2080_Simple_v4 (Autodesk Fusion 360 design; units mm, degrees)
Autodesk Fusion 360 part; units mm, degrees
(part 1 of 2)
sketch "Sketch1" plane through (0, 0, 0) normal (0, 0, 1) x (1, 0, 0)
  line L0 (33.9, 0.2048) -> (33.9, 2.8393) construction
  line L1 (25.5058, -9.8977) -> (25.5381, -9.8746) construction
  arc A0 (33.1214, 8.5414) -> (33.2628, 8.2) centre (33.2628, 8.4) ccw construction
  line L2 (39.9538, 4.5991) -> (39.9678, 4.6363) construction
  line L3 (39.5, 10) -> (38.5, 10) construction
  line L4 (34.9, 10) -> (34.7917, 9.9987) construction
  line L5 (34.4312, 9.8494) -> (34.4022, 9.8222) construction
  line L6 (25.5381, -9.8746) -> (25.5688, -9.8494) construction
  line L7 (25.5978, -9.8222) -> (26.8786, -8.5414) construction
  line L8 (26.7372, -8.2) -> (24.5, -8.2) construction
  line L9 (-38.2, -5.5) -> (-38.2, -3.2628) construction
  line L10 (25.4721, -9.9187) -> (25.5058, -9.8977) construction
  line L11 (38.2, 5.5) -> (38.2, 3.2628) construction
  line L12 (34.5991, 9.9538) -> (34.563, 9.9374) construction
  line L13 (25.5688, -9.8494) -> (25.5978, -9.8222) construction
  line L14 (39.9987, 4.7917) -> (40, 4.8314) construction
  arc A1 (38.2, 3.2628) -> (38.5414, 3.1214) centre (38.4, 3.2628) ccw construction
  arc A2 (-33.1214, -8.5414) -> (-33.2628, -8.2) centre (-33.2628, -8.4) ccw construction
  line L15 (39.9948, 4.7522) -> (39.9987, 4.7917) construction
  arc A3 (26.8786, -8.5414) -> (26.7372, -8.2) centre (26.7372, -8.4) ccw construction
  line L16 (33.6952, 0) -> (33.9, 0.2048) construction
  line L17 (-34.5279, -9.9187) -> (-34.4942, -9.8977) construction
  line L18 (33.9, -0.207) -> (33.6952, 0) construction
  line L19 (-34.563, -9.9374) -> (-34.5279, -9.9187) construction
  line L20 (39.8977, 4.4942) -> (39.9187, 4.5279) construction
  line L21 (32.8393, -3.9) -> (35.5, -6.5607) construction
  line L22 (39.9187, 4.5279) -> (39.9374, 4.563) construction
  line L23 (39.9793, 4.6743) -> (39.9883, 4.713) construction
  line L24 (39.9374, 4.563) -> (39.9538, 4.5991) construction
  line L25 (39.8222, 4.4022) -> (39.8494, 4.4312) construction
  line L26 (33.6952, 0) -> (33.9, 0.2048) construction
  line L27 (39.8494, 4.4312) -> (39.8746, 4.4619) construction
  line L28 (39.9883, 4.713) -> (39.9948, 4.7522) construction
  line L29 (33.9, 2.8393) -> (36.5607, 5.5) construction
  line L30 (38.5414, 3.1214) -> (39.8222, 4.4022) construction
  line L31 (39.8746, 4.4619) -> (39.8977, 4.4942) construction
  line L32 (39.9678, 4.6363) -> (39.9793, 4.6743) construction
  line L33 (-34.4022, -9.8222) -> (-33.1214, -8.5414) construction
  line L34 (36.5607, 5.5) -> (38.2, 5.5) construction
  line L35 (-34.4312, -9.8494) -> (-34.4022, -9.8222) construction
  line L36 (-34.4619, -9.8746) -> (-34.4312, -9.8494) construction
  line L37 (-39.9883, -4.713) -> (-39.9948, -4.7522) construction
  line L38 (-25.4721, -9.9187) -> (-25.437, -9.9374) construction
  line L39 (-39.9538, -4.5991) -> (-39.9678, -4.6363) construction
  line L40 (-39.9678, -4.6363) -> (-39.9793, -4.6743) construction
  line L41 (25.1, -10) -> (25.2083, -9.9987) construction
  line L42 (25.437, 9.9374) -> (25.4009, 9.9538) construction
  line L43 (26.1, -0.207) -> (26.1, -2.8393) construction
  line L44 (25.4009, 9.9538) -> (25.3637, 9.9678) construction
  circle A4 centre (30, 0) radius 2.1 construction
  line L45 (-39.9948, -4.7522) -> (-39.9987, -4.7917) construction
  line L46 (-25.3637, -9.9678) -> (-25.3257, -9.9793) construction
  line L47 (-39.9793, -4.6743) -> (-39.9883, -4.713) construction
  line L48 (26.1, 0.207) -> (26.307, 0) construction
  line L49 (26.1, -2.8393) -> (22.7, -6.2393) construction
  line L50 (30.1999, 3.9) -> (30, 3.7001) construction
  line L51 (26.8786, 8.5414) -> (25.5978, 9.8222) construction
  arc A5 (26.7372, 8.2) -> (26.8786, 8.5414) centre (26.7372, 8.4) ccw construction
  line L52 (-25.437, -9.9374) -> (-25.4009, -9.9538) construction
  line L53 (22.7, 8.2) -> (22.7, 6.2393) construction
  line L54 (-25.5058, -9.8977) -> (-25.4721, -9.9187) construction
  line L55 (25.3637, 9.9678) -> (25.3257, 9.9793) construction
  line L56 (27.1607, 3.9) -> (24.5, 6.5607) construction
  arc A6 (-38.2, -3.2628) -> (-38.5414, -3.1214) centre (-38.4, -3.2628) ccw construction
  line L57 (22.7, -6.2393) -> (22.7, -8.2) construction
  line L58 (24.5, 8.2) -> (26.7372, 8.2) construction
  line L59 (-25.3257, -9.9793) -> (-25.287, -9.9883) construction
  line L60 (-39.9987, -4.7917) -> (-40, -4.8314) construction
  line L61 (-25.287, -9.9883) -> (-25.2478, -9.9948) construction
  line L62 (-25.2478, -9.9948) -> (-25.2083, -9.9987) construction
  line L63 (-25.4009, -9.9538) -> (-25.3637, -9.9678) construction
  line L64 (34.4942, 9.8977) -> (34.4619, 9.8746) construction
  arc A7 (40, 9.5) -> (39.5, 10) centre (39.5, 9.5) ccw construction
  line L65 (40, 8.5) -> (40, 9.5) construction
  line L66 (34.6363, 9.9678) -> (34.5991, 9.9538) construction
  line L67 (-25.2083, -9.9987) -> (-25.1, -10) construction
  line L68 (-39.9374, -4.563) -> (-39.9538, -4.5991) construction
  line L69 (25.2083, -9.9987) -> (25.2478, -9.9948) construction
  line L70 (-39.9187, -4.5279) -> (-39.9374, -4.563) construction
  line L71 (35.5, 8.2) -> (35.5, 6.5607) construction
  line L72 (25.3257, -9.9793) -> (25.3637, -9.9678) construction
  line L73 (33.2628, 8.2) -> (35.5, 8.2) construction
  line L74 (-39.8222, -4.4022) -> (-39.8494, -4.4312) construction
  line L75 (34.4619, 9.8746) -> (34.4312, 9.8494) construction
  line L76 (34.7522, 9.9948) -> (34.713, 9.9883) construction
  line L77 (-39.8494, -4.4312) -> (-39.8746, -4.4619) construction
  line L78 (34.4022, 9.8222) -> (33.1214, 8.5414) construction
  line L79 (34.563, 9.9374) -> (34.5279, 9.9187) construction
  line L80 (34.6743, 9.9793) -> (34.6363, 9.9678) construction
  line L81 (25.287, -9.9883) -> (25.3257, -9.9793) construction
  line L82 (-40, -4.8314) -> (-40, -8.5) construction
  line L83 (34.713, 9.9883) -> (34.6743, 9.9793) construction
  line L84 (-39.8746, -4.4619) -> (-39.8977, -4.4942) construction
  line L85 (25.3637, -9.9678) -> (25.4009, -9.9538) construction
  line L86 (-38.5414, -3.1214) -> (-39.8222, -4.4022) construction
  line L87 (25.4009, -9.9538) -> (25.437, -9.9374) construction
  arc A8 (-26.7372, -8.2) -> (-26.8786, -8.5414) centre (-26.7372, -8.4) ccw construction
  line L88 (38.5, 10) -> (34.9, 10) construction
  line L89 (34.5279, 9.9187) -> (34.4942, 9.8977) construction
  line L90 (34.7917, 9.9987) -> (34.7522, 9.9948) construction
  line L91 (25.437, -9.9374) -> (25.4721, -9.9187) construction
  line L92 (25.2478, -9.9948) -> (25.287, -9.9883) construction
  line L93 (-39.8977, -4.4942) -> (-39.9187, -4.5279) construction
  line L94 (39.9374, -4.563) -> (39.9187, -4.5279) construction
  line L95 (-40, -8.5) -> (-40, -9.5) construction
  line L96 (30, -3.7001) -> (30.1999, -3.9) construction
  line L97 (22.7, -6.2393) -> (22.7, -8.2) construction
  line L98 (24.5, -6.5607) -> (27.1607, -3.9) construction
  line L99 (25.5978, -9.8222) -> (26.8786, -8.5414) construction
  line L100 (25.4721, -9.9187) -> (25.5058, -9.8977) construction
  line L101 (39.8746, -4.4619) -> (39.8494, -4.4312) construction
  line L102 (25.437, -9.9374) -> (25.4721, -9.9187) construction
  line L103 (39.9187, -4.5279) -> (39.8977, -4.4942) construction
  arc A9 (-40, -9.5) -> (-39.5, -10) centre (-39.5, -9.5) ccw construction
  line L104 (24.5, -8.2) -> (24.5, -6.5607) construction
  line L105 (-38.5, -10) -> (-34.8314, -10) construction
  line L106 (39.8222, -4.4022) -> (38.5414, -3.1214) construction
  line L107 (-35.5, -8.2) -> (-35.5, -6.5607) construction
  line L108 (25.3637, -9.9678) -> (25.4009, -9.9538) construction
  line L109 (39.8977, -4.4942) -> (39.8746, -4.4619) construction
  line L110 (26.7372, -8.2) -> (24.5, -8.2) construction
  line L111 (25.287, -9.9883) -> (25.3257, -9.9793) construction
  line L112 (25.4009, -9.9538) -> (25.437, -9.9374) construction
  line L113 (39.8494, -4.4312) -> (39.8222, -4.4022) construction
  arc A10 (26.8786, -8.5414) -> (26.7372, -8.2) centre (26.7372, -8.4) ccw construction
  line L114 (-39.5, -10) -> (-38.5, -10) construction
  line L115 (26.1, -2.8393) -> (22.7, -6.2393) construction
  line L116 (39.9538, -4.5991) -> (39.9374, -4.563) construction
  line L117 (29.8001, -3.9) -> (30, -3.7001) construction
  line L118 (-34.6743, -9.9793) -> (-34.6363, -9.9678) construction
  line L119 (-34.713, -9.9883) -> (-34.6743, -9.9793) construction
  line L120 (33.9, -2.8393) -> (33.9, -0.207) construction
  line L121 (36.5607, -5.5) -> (33.9, -2.8393) construction
  line L122 (25.3257, -9.9793) -> (25.3637, -9.9678) construction
  line L123 (25.2478, -9.9948) -> (25.287, -9.9883) construction
  arc A11 (38.5414, -3.1214) -> (38.2, -3.2628) centre (38.4, -3.2628) ccw construction
  line L124 (25.5058, -9.8977) -> (25.5381, -9.8746) construction
  line L125 (32.8393, 3.9) -> (30.1999, 3.9) construction
  line L126 (-34.7917, -9.9987) -> (-34.7522, -9.9948) construction
  line L127 (25.5381, -9.8746) -> (25.5688, -9.8494) construction
  line L128 (25.1, -10) -> (25.2083, -9.9987) construction
  line L129 (27.1607, -3.9) -> (29.8001, -3.9) construction
  line L130 (-33.2628, -8.2) -> (-35.5, -8.2) construction
  line L131 (35.5, 6.5607) -> (32.8393, 3.9) construction
  line L132 (38.2, -5.5) -> (36.5607, -5.5) construction
  line L133 (-34.7522, -9.9948) -> (-34.713, -9.9883) construction
  line L134 (40, -8.5) -> (40, -4.8314) construction
  line L135 (-34.5991, -9.9538) -> (-34.563, -9.9374) construction
  line L136 (-34.6363, -9.9678) -> (-34.5991, -9.9538) construction
  line L137 (-34.8314, -10) -> (-34.7917, -9.9987) construction
  line L138 (40, 4.8314) -> (40, 8.5) construction
  line L139 (33.9, -0.207) -> (33.6952, 0) construction
  line L140 (25.5978, 9.8222) -> (25.5688, 9.8494) construction
  line L141 (26.307, 0) -> (26.1, -0.207) construction
  line L142 (-33.9, -2.8393) -> (-36.5607, -5.5) construction
  line L143 (24.5, -8.2) -> (24.5, -6.5607) construction
  line L144 (-36.5607, -5.5) -> (-38.2, -5.5) construction
  line L145 (25.3257, 9.9793) -> (25.287, 9.9883) construction
  line L146 (-33.9, -0.207) -> (-33.9, -2.8393) construction
  line L147 (-33.6952, 0) -> (-33.9, -0.207) construction
  line L148 (30, -3.7001) -> (30.1999, -3.9) construction
  line L149 (24.5, 6.5607) -> (24.5, 8.2) construction
  line L150 (30, 3.7001) -> (29.8001, 3.9) construction
  line L151 (-26.8786, -8.5414) -> (-25.5978, -9.8222) construction
  line L152 (25.4721, 9.9187) -> (25.437, 9.9374) construction
  line L153 (26.307, 0) -> (26.1, -0.207) construction
  line L154 (24.5, -6.5607) -> (27.1607, -3.9) construction
  line L155 (25.287, 9.9883) -> (25.2478, 9.9948) construction
  line L156 (26.1, 2.8393) -> (26.1, 0.207) construction
  line L157 (27.1607, -3.9) -> (29.8001, -3.9) construction
  line L158 (25.5688, 9.8494) -> (25.5381, 9.8746) construction
  line L159 (-25.5978, -9.8222) -> (-25.5688, -9.8494) construction
  line L160 (25.2083, 9.9987) -> (25.1, 10) construction
  line L161 (29.8001, -3.9) -> (30, -3.7001) construction
  line L162 (26.1, 0.207) -> (26.307, 0) construction
  line L163 (-25.5688, -9.8494) -> (-25.5381, -9.8746) construction
  line L164 (-33.9, 0.2048) -> (-33.6952, 0) construction
  line L165 (25.2478, 9.9948) -> (25.2083, 9.9987) construction
  line L166 (30.1999, -3.9) -> (32.8393, -3.9) construction
  line L167 (-24.5, -8.2) -> (-26.7372, -8.2) construction
  line L168 (22.7, 6.2393) -> (26.1, 2.8393) construction
  line L169 (25.5381, 9.8746) -> (25.5058, 9.8977) construction
  line L170 (25.5058, 9.8977) -> (25.4721, 9.9187) construction
  line L171 (29.8001, 3.9) -> (27.1607, 3.9) construction
  line L172 (-35.5, -6.5607) -> (-32.8393, -3.9) construction
  line L173 (39.9793, 4.6743) -> (39.9883, 4.713) construction
  line L174 (-22.7, -6.2393) -> (-26.1, -2.8393) construction
  line L175 (39.9883, 4.713) -> (39.9948, 4.7522) construction
  line L176 (39.9987, 4.7917) -> (40, 4.8314) construction
  line L177 (40, 4.8314) -> (40, 8.5) construction
  line L178 (39.9948, 4.7522) -> (39.9987, 4.7917) construction
  line L179 (14.5991, -9.9538) -> (14.6363, -9.9678) construction
  line L180 (10.1999, -3.9) -> (12.8393, -3.9) construction
  line L181 (-26.307, 0) -> (-26.1, 0.207) construction
  line L182 (13.9, -2.8393) -> (13.9, -0.207) construction
  line L183 (14.7917, -9.9987) -> (14.9, -10) construction
  arc A12 (38.2, 3.2628) -> (38.5414, 3.1214) centre (38.4, 3.2628) ccw construction
  line L184 (14.4619, -9.8746) -> (14.4942, -9.8977) construction
  line L185 (35.5, 6.5607) -> (32.8393, 3.9) construction
  line L186 (14.6363, -9.9678) -> (14.6743, -9.9793) construction
  line L187 (12.8393, 3.9) -> (10.1999, 3.9) construction
  line L188 (15.5, -6.5607) -> (15.5, -8.2) construction
  line L189 (13.9, 0.207) -> (13.9, 2.8393) construction
  line L190 (-26.1, -2.8393) -> (-26.1, -0.207) construction
  circle A13 centre (-30, 0) radius 2.1 construction
  line L191 (12.8393, -3.9) -> (15.5, -6.5607) construction
  line L192 (13.693, 0) -> (13.9, 0.207) construction
  line L193 (14.713, -9.9883) -> (14.7522, -9.9948) construction
  line L194 (13.9, 2.8393) -> (17.3, 6.2393) construction
  line L195 (-26.1, -0.207) -> (-26.307, 0) construction
  line L196 (26.8786, 8.5414) -> (25.5978, 9.8222) construction
  line L197 (25.5978, 9.8222) -> (25.5688, 9.8494) construction
  line L198 (-25.5381, 9.8746) -> (-25.5688, 9.8494) construction
  line L199 (-25.5058, 9.8977) -> (-25.5381, 9.8746) construction
  circle A14 centre (-10, 0) radius 2.1 construction
  line L200 (-14.4942, 9.8977) -> (-14.5279, 9.9187) construction
  line L201 (-7.1607, -3.9) -> (-4.5, -6.5607) construction
  line L202 (-14.5991, 9.9538) -> (-14.6363, 9.9678) construction
  line L203 (-13.1214, 8.5414) -> (-14.4022, 9.8222) construction
  line L204 (-14.5279, 9.9187) -> (-14.563, 9.9374) construction
  line L205 (4.5, -8.2) -> (4.5, -6.5607) construction
  line L206 (-6.1, -2.8393) -> (-6.1, -0.207) construction
  line L207 (-5.5058, -9.8977) -> (-5.4721, -9.9187) construction
  line L208 (6.1, 2.8393) -> (6.1, 0.207) construction
  line L209 (-14.713, 9.9883) -> (-14.7522, 9.9948) construction
  line L210 (-14.6363, 9.9678) -> (-14.6743, 9.9793) construction
  line L211 (-10, -3.7001) -> (-9.8001, -3.9) construction
  line L212 (-5.4009, -9.9538) -> (-5.3637, -9.9678) construction
  line L213 (7.1607, 3.9) -> (4.5, 6.5607) construction
  line L214 (9.8001, 3.9) -> (7.1607, 3.9) construction
  line L215 (-2.7, -6.2393) -> (-6.1, -2.8393) construction
  line L216 (-6.1, -2.8393) -> (-6.1, -0.207) construction
  line L217 (-10.1999, -3.9) -> (-10, -3.7001) construction
  line L218 (10, 3.7001) -> (9.8001, 3.9) construction
  line L219 (-9.8001, -3.9) -> (-7.1607, -3.9) construction
  line L220 (-6.307, 0) -> (-6.1, 0.207) construction
  line L221 (10.1999, 3.9) -> (10, 3.7001) construction
  line L222 (-14.4022, 9.8222) -> (-14.4312, 9.8494) construction
  line L223 (-5.5381, -9.8746) -> (-5.5058, -9.8977) construction
  line L224 (-6.1, -0.207) -> (-6.307, 0) construction
  line L225 (2.7, 6.2393) -> (6.1, 2.8393) construction
  line L226 (-14.4312, 9.8494) -> (-14.4619, 9.8746) construction
  line L227 (-10.1999, -3.9) -> (-10, -3.7001) construction
  line L228 (-5.5688, -9.8494) -> (-5.5381, -9.8746) construction
  line L229 (-14.7522, 9.9948) -> (-14.7917, 9.9987) construction
  line L230 (-12.8393, 3.9) -> (-15.5, 6.5607) construction
  line L231 (-14.7917, 9.9987) -> (-14.9, 10) construction
  arc A15 (-6.7372, -8.2) -> (-6.8786, -8.5414) centre (-6.7372, -8.4) ccw construction
  line L232 (-14.4619, 9.8746) -> (-14.4942, 9.8977) construction
  line L233 (-5.3257, -9.9793) -> (-5.287, -9.9883) construction
  line L234 (6.1, 0.207) -> (6.307, 0) construction
  line L235 (-5.287, -9.9883) -> (-5.2478, -9.9948) construction
  line L236 (10, -3.7001) -> (10.1999, -3.9) construction
  line L237 (-5.4009, -9.9538) -> (-5.3637, -9.9678) construction
  line L238 (-15.5, 6.5607) -> (-15.5, 8.2) construction
  line L239 (-5.437, -9.9374) -> (-5.4009, -9.9538) construction
  line L240 (-15.5, 8.2) -> (-13.2628, 8.2) construction
  circle A16 centre (10, 0) radius 2.1 construction
  line L241 (-17.3, 6.2393) -> (-13.9, 2.8393) construction
  line L242 (2.7, -6.2393) -> (2.7, -8.2) construction
  line L243 (-5.2478, -9.9948) -> (-5.2083, -9.9987) construction
  line L244 (9.8001, -3.9) -> (10, -3.7001) construction
  line L245 (-15.5, -6.5607) -> (-12.8393, -3.9) construction
  line L246 (-17.3, 8.2) -> (-17.3, 6.2393) construction
  line L247 (6.1, -2.8393) -> (2.7, -6.2393) construction
  line L248 (-5.2083, -9.9987) -> (-5.1, -10) construction
  line L249 (-14.563, 9.9374) -> (-14.5991, 9.9538) construction
  line L250 (6.1, -0.207) -> (6.1, -2.8393) construction
  line L251 (-14.6743, 9.9793) -> (-14.713, 9.9883) construction
  arc A17 (-13.2628, 8.2) -> (-13.1214, 8.5414) centre (-13.2628, 8.4) ccw construction
  line L252 (6.307, 0) -> (6.1, -0.207) construction
  line L253 (-5.3637, -9.9678) -> (-5.3257, -9.9793) construction
  arc A18 (-13.1214, -8.5414) -> (-13.2628, -8.2) centre (-13.2628, -8.4) ccw construction
  line L254 (-14.4022, -9.8222) -> (-13.1214, -8.5414) construction
  arc A19 (6.8786, -8.5414) -> (6.7372, -8.2) centre (6.7372, -8.4) ccw construction
  line L255 (-14.5991, -9.9538) -> (-14.563, -9.9374) construction
  line L256 (-13.9, -2.8393) -> (-17.3, -6.2393) construction
  line L257 (4.5, -6.5607) -> (7.1607, -3.9) construction
  line L258 (-5.5058, -9.8977) -> (-5.4721, -9.9187) construction
  line L259 (-14.7522, -9.9948) -> (-14.713, -9.9883) construction
  line L260 (-5.5688, -9.8494) -> (-5.5381, -9.8746) construction
  line L261 (-13.9, -0.207) -> (-13.9, -2.8393) construction
  line L262 (-13.2628, -8.2) -> (-15.5, -8.2) construction
  line L263 (5.5381, -9.8746) -> (5.5688, -9.8494) construction
  line L264 (-14.5279, -9.9187) -> (-14.4942, -9.8977) construction
  line L265 (-14.9, -10) -> (-14.7917, -9.9987) construction
  line L266 (6.7372, -8.2) -> (4.5, -8.2) construction
  line L267 (-14.6743, -9.9793) -> (-14.6363, -9.9678) construction
  line L268 (-4.5, -8.2) -> (-6.7372, -8.2) construction
  line L269 (-15.5, -8.2) -> (-15.5, -6.5607) construction
  line L270 (-14.4312, -9.8494) -> (-14.4022, -9.8222) construction
  line L271 (-17.3, -6.2393) -> (-17.3, -8.2) construction
  line L272 (-5.5381, -9.8746) -> (-5.5058, -9.8977) construction
  line L273 (-14.713, -9.9883) -> (-14.6743, -9.9793) construction
  line L274 (-13.9, 0.207) -> (-13.693, 0) construction
  line L275 (-13.693, 0) -> (-13.9, -0.207) construction
  line L276 (-14.4942, -9.8977) -> (-14.4619, -9.8746) construction
  line L277 (5.5688, -9.8494) -> (5.5978, -9.8222) construction
  line L278 (-5.4721, -9.9187) -> (-5.437, -9.9374) construction
  line L279 (7.1607, -3.9) -> (9.8001, -3.9) construction
  line L280 (-6.8786, -8.5414) -> (-5.5978, -9.8222) construction
  line L281 (-14.4619, -9.8746) -> (-14.4312, -9.8494) construction
  line L282 (-14.563, -9.9374) -> (-14.5279, -9.9187) construction
  line L283 (-14.7917, -9.9987) -> (-14.7522, -9.9948) construction
  line L284 (-5.5978, -9.8222) -> (-5.5688, -9.8494) construction
  line L285 (5.5978, -9.8222) -> (6.8786, -8.5414) construction
  line L286 (-4.5, -6.5607) -> (-4.5, -8.2) construction
  line L287 (-14.6363, -9.9678) -> (-14.5991, -9.9538) construction
  line L288 (-26.1, -0.207) -> (-26.307, 0) construction
  line L289 (-5.1, -10) -> (5.1, -10) construction
  line L290 (-13.9, 2.8393) -> (-13.9, 0.207) construction
  line L291 (5.4721, -9.9187) -> (5.5058, -9.8977) construction
  line L292 (5.437, -9.9374) -> (5.4721, -9.9187) construction
  line L293 (5.5058, -9.8977) -> (5.5381, -9.8746) construction
  line L294 (5.3257, -9.9793) -> (5.3637, -9.9678) construction
  line L295 (-15.5, 8.2) -> (-13.2628, 8.2) construction
  line L296 (5.4009, -9.9538) -> (5.437, -9.9374) construction
  line L297 (-10.1999, 3.9) -> (-12.8393, 3.9) construction
  line L298 (-2.7, -6.2393) -> (-6.1, -2.8393) construction
  arc A20 (-26.8786, 8.5414) -> (-26.7372, 8.2) centre (-26.7372, 8.4) ccw construction
  line L299 (-10.1999, 3.9) -> (-12.8393, 3.9) construction
  line L300 (5.2083, -9.9987) -> (5.2478, -9.9948) construction
  line L301 (2.7, -8.2) -> (-2.7, -8.2) construction
  circle A21 centre (-10, 0) radius 2.1 construction
  line L302 (-2.7, -8.2) -> (-2.7, -6.2393) construction
  line L303 (-22.7, 6.2393) -> (-22.7, 8.2) construction
  line L304 (-26.1, 0.207) -> (-26.1, 2.8393) construction
  line L305 (-13.1214, 8.5414) -> (-14.4022, 9.8222) construction
  line L306 (-14.4022, 9.8222) -> (-14.4312, 9.8494) construction
  line L307 (-25.2083, 9.9987) -> (-25.2478, 9.9948) construction
  line L308 (-24.5, 8.2) -> (-24.5, 6.5607) construction
  line L309 (-26.307, 0) -> (-26.1, 0.207) construction
  line L310 (-29.8001, 3.9) -> (-30, 3.7001) construction
  line L311 (5.3637, -9.9678) -> (5.4009, -9.9538) construction
  line L312 (-12.8393, -3.9) -> (-10.1999, -3.9) construction
  line L313 (5.2478, -9.9948) -> (5.287, -9.9883) construction
  line L314 (5.287, -9.9883) -> (5.3257, -9.9793) construction
  line L315 (-12.8393, 3.9) -> (-15.5, 6.5607) construction
  line L316 (5.1, -10) -> (5.2083, -9.9987) construction
  line L317 (-6.1, -0.207) -> (-6.307, 0) construction
  line L318 (-6.7372, 8.2) -> (-4.5, 8.2) construction
  line L319 (-10, 3.7001) -> (-10.1999, 3.9) construction
  line L320 (-2.7, 6.2393) -> (-2.7, 8.2) construction
  line L321 (-5.5978, 9.8222) -> (-6.8786, 8.5414) construction
  line L322 (-5.5978, 9.8222) -> (-6.8786, 8.5414) construction
  line L323 (-5.2478, 9.9948) -> (-5.287, 9.9883) construction
  line L324 (-5.5058, 9.8977) -> (-5.5381, 9.8746) construction
  line L325 (-5.5058, 9.8977) -> (-5.5381, 9.8746) construction
  arc A22 (-6.8786, 8.5414) -> (-6.7372, 8.2) centre (-6.7372, 8.4) ccw construction
  line L326 (-5.5688, 9.8494) -> (-5.5978, 9.8222) construction
  line L327 (-5.5688, 9.8494) -> (-5.5978, 9.8222) construction
  line L328 (-5.5381, 9.8746) -> (-5.5688, 9.8494) construction
  line L329 (-5.1, 10) -> (-5.2083, 9.9987) construction
  line L330 (-9.8001, 3.9) -> (-10, 3.7001) construction
  line L331 (-5.287, 9.9883) -> (-5.3257, 9.9793) construction
  arc A23 (6.7372, 8.2) -> (6.8786, 8.5414) centre (6.7372, 8.4) ccw construction
  line L332 (-5.3257, 9.9793) -> (-5.3637, 9.9678) construction
  line L333 (-5.2083, 9.9987) -> (-5.2478, 9.9948) construction
  line L334 (-4.5, 6.5607) -> (-7.1607, 3.9) construction
  arc A24 (-6.8786, 8.5414) -> (-6.7372, 8.2) centre (-6.7372, 8.4) ccw construction
  line L335 (-6.1, 2.8393) -> (-2.7, 6.2393) construction
  line L336 (-5.4009, 9.9538) -> (-5.437, 9.9374) construction
  line L337 (-5.437, 9.9374) -> (-5.4721, 9.9187) construction
  line L338 (-5.2083, 9.9987) -> (-5.2478, 9.9948) construction
  line L339 (-6.307, 0) -> (-6.1, 0.207) construction
  line L340 (-5.4721, 9.9187) -> (-5.5058, 9.8977) construction
  line L341 (-5.437, 9.9374) -> (-5.4721, 9.9187) construction
  line L342 (-5.4009, 9.9538) -> (-5.437, 9.9374) construction
  line L343 (-6.7372, 8.2) -> (-4.5, 8.2) construction
  line L344 (-6.1, 0.207) -> (-6.1, 2.8393) construction
  line L345 (2.7, 8.2) -> (2.7, 6.2393) construction
  line L346 (-5.3257, 9.9793) -> (-5.3637, 9.9678) construction
  line L347 (-2.7, 8.2) -> (2.7, 8.2) construction
  line L348 (-5.287, 9.9883) -> (-5.3257, 9.9793) construction
  line L349 (4.5, 6.5607) -> (4.5, 8.2) construction
  line L350 (-7.1607, 3.9) -> (-9.8001, 3.9) construction
  line L351 (5.2083, 9.9987) -> (5.1, 10) construction
  line L352 (-5.3637, 9.9678) -> (-5.4009, 9.9538) construction
  line L353 (-5.3637, 9.9678) -> (-5.4009, 9.9538) construction
  line L354 (5.2478, 9.9948) -> (5.2083, 9.9987) construction
  line L355 (-5.2478, 9.9948) -> (-5.287, 9.9883) construction
  line L356 (-5.5381, 9.8746) -> (-5.5688, 9.8494) construction
  line L357 (-5.1, 10) -> (-5.2083, 9.9987) construction
  line L358 (5.287, 9.9883) -> (5.2478, 9.9948) construction
  arc A25 (-6.7372, -8.2) -> (-6.8786, -8.5414) centre (-6.7372, -8.4) ccw construction
  line L359 (5.437, 9.9374) -> (5.4009, 9.9538) construction
  line L360 (-5.287, -9.9883) -> (-5.2478, -9.9948) construction
  line L361 (-4.5, 8.2) -> (-4.5, 6.5607) construction
  line L362 (-5.3637, -9.9678) -> (-5.3257, -9.9793) construction
  line L363 (-5.4721, 9.9187) -> (-5.5058, 9.8977) construction
  line L364 (-9.8001, -3.9) -> (-7.1607, -3.9) construction
  line L365 (5.3637, 9.9678) -> (5.3257, 9.9793) construction
  line L366 (-9.8001, 3.9) -> (-10, 3.7001) construction
  line L367 (6.8786, 8.5414) -> (5.5978, 9.8222) construction
  line L368 (-4.5, -6.5607) -> (-4.5, -8.2) construction
  line L369 (-4.5, 8.2) -> (-4.5, 6.5607) construction
  line L370 (-2.7, -8.2) -> (-2.7, -6.2393) construction
  line L371 (-7.1607, 3.9) -> (-9.8001, 3.9) construction
  line L372 (-4.5, -8.2) -> (-6.7372, -8.2) construction
  line L373 (5.5058, 9.8977) -> (5.4721, 9.9187) construction
  line L374 (-10, 3.7001) -> (-10.1999, 3.9) construction
  line L375 (5.5381, 9.8746) -> (5.5058, 9.8977) construction
  line L376 (-5.2478, -9.9948) -> (-5.2083, -9.9987) construction
  line L377 (-6.1, 0.207) -> (-6.1, 2.8393) construction
  line L378 (5.4721, 9.9187) -> (5.437, 9.9374) construction
  line L379 (-4.5, 6.5607) -> (-7.1607, 3.9) construction
  line L380 (-5.5978, -9.8222) -> (-5.5688, -9.8494) construction
  line L381 (-5.437, -9.9374) -> (-5.4009, -9.9538) construction
  line L382 (5.5978, 9.8222) -> (5.5688, 9.8494) construction
  line L383 (5.4009, 9.9538) -> (5.3637, 9.9678) construction
  line L384 (5.3257, 9.9793) -> (5.287, 9.9883) construction
  line L385 (-5.2083, -9.9987) -> (-5.1, -10) construction
  line L386 (-5.3257, -9.9793) -> (-5.287, -9.9883) construction
  line L387 (5.5688, 9.8494) -> (5.5381, 9.8746) construction
  line L388 (4.5, 8.2) -> (6.7372, 8.2) construction
  line L389 (-2.7, 6.2393) -> (-2.7, 8.2) construction
  line L390 (-6.8786, -8.5414) -> (-5.5978, -9.8222) construction
  line L391 (-5.4721, -9.9187) -> (-5.437, -9.9374) construction
  line L392 (-6.1, 2.8393) -> (-2.7, 6.2393) construction
  line L393 (5.1, 10) -> (-5.1, 10) construction
  line L394 (-10, -3.7001) -> (-9.8001, -3.9) construction
  line L395 (-7.1607, -3.9) -> (-4.5, -6.5607) construction
  line L396 (39.8977, -4.4942) -> (39.8746, -4.4619) construction
  arc A26 (38.5414, -3.1214) -> (38.2, -3.2628) centre (38.4, -3.2628) ccw construction
  line L397 (39.9948, -4.7522) -> (39.9883, -4.713) construction
  arc A27 (33.2628, -8.2) -> (33.1214, -8.5414) centre (33.2628, -8.4) ccw construction
  line L398 (39.9374, -4.563) -> (39.9187, -4.5279) construction
  line L399 (39.8746, -4.4619) -> (39.8494, -4.4312) construction
  line L400 (38.2, -3.2628) -> (38.2, -5.5) construction
  line L401 (34.6363, -9.9678) -> (34.6743, -9.9793) construction
  line L402 (39.9987, -4.7917) -> (39.9948, -4.7522) construction
  line L403 (38.2, -3.2628) -> (38.2, -5.5) construction
  line L404 (32.8393, -3.9) -> (35.5, -6.5607) construction
  line L405 (25.5688, -9.8494) -> (25.5978, -9.8222) construction
  line L406 (38.2, -5.5) -> (36.5607, -5.5) construction
  line L407 (39.9948, -4.7522) -> (39.9883, -4.713) construction
  line L408 (40, -4.8314) -> (39.9987, -4.7917) construction
  line L409 (25.2083, -9.9987) -> (25.2478, -9.9948) construction
  line L410 (39.9678, -4.6363) -> (39.9538, -4.5991) construction
  line L411 (34.713, -9.9883) -> (34.7522, -9.9948) construction
  line L412 (40, -4.8314) -> (39.9987, -4.7917) construction
  line L413 (34.5279, -9.9187) -> (34.563, -9.9374) construction
  line L414 (39.9793, -4.6743) -> (39.9678, -4.6363) construction
  line L415 (36.5607, -5.5) -> (33.9, -2.8393) construction
  line L416 (39.9987, -4.7917) -> (39.9948, -4.7522) construction
  line L417 (-5.1, -10) -> (5.1, -10) construction
  line L418 (34.7522, -9.9948) -> (34.7917, -9.9987) construction
  line L419 (39.9187, -4.5279) -> (39.8977, -4.4942) construction
  line L420 (39.8494, -4.4312) -> (39.8222, -4.4022) construction
  line L421 (39.9538, -4.5991) -> (39.9374, -4.563) construction
  line L422 (39.9883, -4.713) -> (39.9793, -4.6743) construction
  line L423 (34.7917, -9.9987) -> (34.8314, -10) construction
  line L424 (39.9678, -4.6363) -> (39.9538, -4.5991) construction
  line L425 (39.8222, -4.4022) -> (38.5414, -3.1214) construction
  line L426 (34.6743, -9.9793) -> (34.713, -9.9883) construction
  line L427 (39.9793, -4.6743) -> (39.9678, -4.6363) construction
  line L428 (39.9883, -4.713) -> (39.9793, -4.6743) construction
  line L429 (34.5991, -9.9538) -> (34.6363, -9.9678) construction
  line L430 (34.563, -9.9374) -> (34.5991, -9.9538) construction
  line L431 (40, -9.5) -> (40, -8.5) construction
  line L432 (-2.7, 8.2) -> (2.7, 8.2) construction
  line L433 (34.6743, -9.9793) -> (34.713, -9.9883) construction
  line L434 (34.8314, -10) -> (38.5, -10) construction
  line L435 (34.5991, -9.9538) -> (34.6363, -9.9678) construction
  line L436 (34.4022, -9.8222) -> (34.4312, -9.8494) construction
  line L437 (38.5, -10) -> (39.5, -10) construction
  line L438 (34.563, -9.9374) -> (34.5991, -9.9538) construction
  line L439 (34.7917, -9.9987) -> (34.8314, -10) construction
  line L440 (40, -8.5) -> (40, -4.8314) construction
  line L441 (35.5, -8.2) -> (33.2628, -8.2) construction
  line L442 (34.4619, -9.8746) -> (34.4942, -9.8977) construction
  line L443 (34.4312, -9.8494) -> (34.4619, -9.8746) construction
  line L444 (33.1214, -8.5414) -> (34.4022, -9.8222) construction
  line L445 (34.7522, -9.9948) -> (34.7917, -9.9987) construction
  line L446 (34.4312, -9.8494) -> (34.4619, -9.8746) construction
  line L447 (34.8314, -10) -> (38.5, -10) construction
  line L448 (40, -9.5) -> (40, -8.5) construction
  line L449 (33.1214, -8.5414) -> (34.4022, -9.8222) construction
  arc A28 (39.5, -10) -> (40, -9.5) centre (39.5, -9.5) ccw construction
  line L450 (34.6363, -9.9678) -> (34.6743, -9.9793) construction
  line L451 (34.4619, -9.8746) -> (34.4942, -9.8977) construction
  line L452 (34.4022, -9.8222) -> (34.4312, -9.8494) construction
  line L453 (35.5, -6.5607) -> (35.5, -8.2) construction
  line L454 (34.4942, -9.8977) -> (34.5279, -9.9187) construction
  arc A29 (39.5, -10) -> (40, -9.5) centre (39.5, -9.5) ccw construction
  line L455 (30.1999, -3.9) -> (32.8393, -3.9) construction
  line L456 (34.4942, -9.8977) -> (34.5279, -9.9187) construction
  arc A30 (33.2628, -8.2) -> (33.1214, -8.5414) centre (33.2628, -8.4) ccw construction
  line L457 (35.5, -6.5607) -> (35.5, -8.2) construction
  line L458 (34.5279, -9.9187) -> (34.563, -9.9374) construction
  circle A31 centre (30, 0) radius 2.1 construction
  line L459 (33.9, -2.8393) -> (33.9, -0.207) construction
  line L460 (26.1, -0.207) -> (26.1, -2.8393) construction
  line L461 (25.1, 10) -> (14.9, 10) construction
  line L462 (14.9, -10) -> (25.1, -10) construction
  line L463 (17.3, 8.2) -> (22.7, 8.2) construction
  line L464 (38.5, -10) -> (39.5, -10) construction
  line L465 (2.7, -8.2) -> (-2.7, -8.2) construction
  line L466 (35.5, -8.2) -> (33.2628, -8.2) construction
  line L467 (34.713, -9.9883) -> (34.7522, -9.9948) construction
  line L468 (5.1, 10) -> (-5.1, 10) construction
  line L469 (22.7, -8.2) -> (17.3, -8.2) construction
  line L470 (12.8393, -3.9) -> (15.5, -6.5607) construction
  line L471 (-14.4942, -9.8977) -> (-14.4619, -9.8746) construction
  line L472 (-36.5607, 5.5) -> (-33.9, 2.8393) construction
  line L473 (-39.9987, 4.7917) -> (-39.9948, 4.7522) construction
  line L474 (-39.9187, 4.5279) -> (-39.8977, 4.4942) construction
  line L475 (-38.2, 5.5) -> (-36.5607, 5.5) construction
  line L476 (13.9, -2.8393) -> (13.9, -0.207) construction
  line L477 (10.1999, -3.9) -> (12.8393, -3.9) construction
  line L478 (-39.8977, 4.4942) -> (-39.8746, 4.4619) construction
  line L479 (13.9, -0.207) -> (13.693, 0) construction
  line L480 (-33.9, 2.8393) -> (-33.9, 0.2048) construction
  arc A32 (-13.1214, -8.5414) -> (-13.2628, -8.2) centre (-13.2628, -8.4) ccw construction
  line L481 (-14.4022, -9.8222) -> (-13.1214, -8.5414) construction
  line L482 (-38.2, 3.2628) -> (-38.2, 5.5) construction
  line L483 (13.693, 0) -> (13.9, 0.207) construction
  line L484 (-39.9374, 4.563) -> (-39.9187, 4.5279) construction
  line L485 (-39.8222, 4.4022) -> (-38.5414, 3.1214) construction
  line L486 (-14.4312, -9.8494) -> (-14.4022, -9.8222) construction
  line L487 (-13.2628, -8.2) -> (-15.5, -8.2) construction
  line L488 (-33.9, 0.2048) -> (-33.6952, 0) construction
  line L489 (-39.8746, 4.4619) -> (-39.8494, 4.4312) construction
  line L490 (-39.9678, 4.6363) -> (-39.9538, 4.5991) construction
  line L491 (-14.4619, -9.8746) -> (-14.4312, -9.8494) construction
  line L492 (-33.6952, 0) -> (-33.9, -0.207) construction
  line L493 (-39.8494, 4.4312) -> (-39.8222, 4.4022) construction
  line L494 (14.713, -9.9883) -> (14.7522, -9.9948) construction
  line L495 (-14.563, -9.9374) -> (-14.5279, -9.9187) construction
  line L496 (-40, 8.5) -> (-40, 4.8314) construction
  line L497 (14.6743, -9.9793) -> (14.713, -9.9883) construction
  arc A33 (-26.7372, -8.2) -> (-26.8786, -8.5414) centre (-26.7372, -8.4) ccw construction
  line L498 (-25.4721, -9.9187) -> (-25.437, -9.9374) construction
  line L499 (-39.9793, 4.6743) -> (-39.9678, 4.6363) construction
  line L500 (-14.5279, -9.9187) -> (-14.4942, -9.8977) construction
  line L501 (-30.1999, -3.9) -> (-30, -3.7001) construction
  line L502 (-22.7, -8.2) -> (-22.7, -6.2393) construction
  line L503 (-25.2083, -9.9987) -> (-25.1, -10) construction
  line L504 (14.563, -9.9374) -> (14.5991, -9.9538) construction
  line L505 (14.6363, -9.9678) -> (14.6743, -9.9793) construction
  line L506 (-30, -3.7001) -> (-29.8001, -3.9) construction
  line L507 (14.5991, -9.9538) -> (14.6363, -9.9678) construction
  line L508 (-32.8393, 3.9) -> (-35.5, 6.5607) construction
  line L509 (-30.1999, 3.9) -> (-32.8393, 3.9) construction
  line L510 (14.7522, -9.9948) -> (14.7917, -9.9987) construction
  line L511 (-14.7522, -9.9948) -> (-14.713, -9.9883) construction
  line L512 (-25.5058, -9.8977) -> (-25.4721, -9.9187) construction
  line L513 (-14.6363, -9.9678) -> (-14.5991, -9.9538) construction
  line L514 (-40, 4.8314) -> (-39.9987, 4.7917) construction
  line L515 (-14.7917, -9.9987) -> (-14.7522, -9.9948) construction
  line L516 (-25.4009, -9.9538) -> (-25.3637, -9.9678) construction
  line L517 (-14.9, -10) -> (-14.7917, -9.9987) construction
  arc A34 (13.2628, -8.2) -> (13.1214, -8.5414) centre (13.2628, -8.4) ccw construction
  line L518 (-14.5991, -9.9538) -> (-14.563, -9.9374) construction
  line L519 (14.7917, -9.9987) -> (14.9, -10) construction
  line L520 (-14.6743, -9.9793) -> (-14.6363, -9.9678) construction
  line L521 (-14.713, -9.9883) -> (-14.6743, -9.9793) construction
  line L522 (-25.287, -9.9883) -> (-25.2478, -9.9948) construction
  line L523 (14.5279, -9.9187) -> (14.563, -9.9374) construction
  line L524 (-25.5688, -9.8494) -> (-25.5381, -9.8746) construction
  line L525 (-22.7, -6.2393) -> (-26.1, -2.8393) construction
  line L526 (-25.2478, -9.9948) -> (-25.2083, -9.9987) construction
  line L527 (14.4022, -9.8222) -> (14.4312, -9.8494) construction
  line L528 (15.5, -8.2) -> (13.2628, -8.2) construction
  line L529 (-25.3257, -9.9793) -> (-25.287, -9.9883) construction
  line L530 (-13.9, -2.8393) -> (-17.3, -6.2393) construction
  line L531 (-24.5, -8.2) -> (-26.7372, -8.2) construction
  line L532 (-27.1607, -3.9) -> (-24.5, -6.5607) construction
  line L533 (-25.437, -9.9374) -> (-25.4009, -9.9538) construction
  line L534 (-25.1, -10) -> (-14.9, -10) construction
  line L535 (-26.8786, -8.5414) -> (-25.5978, -9.8222) construction
  line L536 (14.4619, -9.8746) -> (14.4942, -9.8977) construction
  line L537 (13.1214, -8.5414) -> (14.4022, -9.8222) construction
  line L538 (-24.5, -6.5607) -> (-24.5, -8.2) construction
  line L539 (14.4942, -9.8977) -> (14.5279, -9.9187) construction
  line L540 (-17.3, -6.2393) -> (-17.3, -8.2) construction
  line L541 (-25.5978, -9.8222) -> (-25.5688, -9.8494) construction
  line L542 (-15.5, -8.2) -> (-15.5, -6.5607) construction
  line L543 (-17.3, -8.2) -> (-22.7, -8.2) construction
  line L544 (-29.8001, -3.9) -> (-27.1607, -3.9) construction
  line L545 (-25.3637, -9.9678) -> (-25.3257, -9.9793) construction
  line L546 (14.4312, -9.8494) -> (14.4619, -9.8746) construction
  line L547 (-25.4009, 9.9538) -> (-25.437, 9.9374) construction
  line L548 (-25.2478, 9.9948) -> (-25.287, 9.9883) construction
  line L549 (-39.9538, -4.5991) -> (-39.9678, -4.6363) construction
  line L550 (-33.9, -2.8393) -> (-36.5607, -5.5) construction
  line L551 (-25.2083, 9.9987) -> (-25.2478, 9.9948) construction
  line L552 (-39.8494, -4.4312) -> (-39.8746, -4.4619) construction
  line L553 (-38.5414, -3.1214) -> (-39.8222, -4.4022) construction
  line L554 (-39.9374, -4.563) -> (-39.9538, -4.5991) construction
  line L555 (24.5, 8.2) -> (26.7372, 8.2) construction
  line L556 (-39.9987, -4.7917) -> (-40, -4.8314) construction
  line L557 (22.7, -8.2) -> (17.3, -8.2) construction
  line L558 (15.5, -6.5607) -> (15.5, -8.2) construction
  line L559 (-25.287, 9.9883) -> (-25.3257, 9.9793) construction
  line L560 (-25.4721, 9.9187) -> (-25.5058, 9.8977) construction
  line L561 (-39.8977, -4.4942) -> (-39.9187, -4.5279) construction
  line L562 (17.3, -8.2) -> (17.3, -6.2393) construction
  line L563 (14.9, -10) -> (25.1, -10) construction
  line L564 (-39.9793, -4.6743) -> (-39.9883, -4.713) construction
  line L565 (-25.1, 10) -> (-25.2083, 9.9987) construction
  line L566 (-38.2, -5.5) -> (-38.2, -3.2628) construction
  line L567 (-25.3257, 9.9793) -> (-25.3637, 9.9678) construction
  arc A35 (-38.2, -3.2628) -> (-38.5414, -3.1214) centre (-38.4, -3.2628) ccw construction
  line L568 (-35.5, -6.5607) -> (-32.8393, -3.9) construction
  line L569 (-39.9883, -4.713) -> (-39.9948, -4.7522) construction
  line L570 (-39.8222, -4.4022) -> (-39.8494, -4.4312) construction
  line L571 (17.3, -6.2393) -> (13.9, -2.8393) construction
  line L572 (-39.8746, -4.4619) -> (-39.8977, -4.4942) construction
  line L573 (-25.3637, 9.9678) -> (-25.4009, 9.9538) construction
  line L574 (-39.9948, -4.7522) -> (-39.9987, -4.7917) construction
  line L575 (-39.9678, -4.6363) -> (-39.9793, -4.6743) construction
  line L576 (-36.5607, -5.5) -> (-38.2, -5.5) construction
  line L577 (-25.437, 9.9374) -> (-25.4721, 9.9187) construction
  line L578 (-39.9187, -4.5279) -> (-39.9374, -4.563) construction
  line L579 (-26.1, 2.8393) -> (-22.7, 6.2393) construction
  line L580 (14.7522, 9.9948) -> (14.713, 9.9883) construction
  line L581 (-26.7372, 8.2) -> (-24.5, 8.2) construction
  line L582 (-27.1607, 3.9) -> (-29.8001, 3.9) construction
  line L583 (14.7917, 9.9987) -> (14.7522, 9.9948) construction
  line L584 (-14.563, 9.9374) -> (-14.5991, 9.9538) construction
  line L585 (-25.5381, 9.8746) -> (-25.5688, 9.8494) construction
  line L586 (-14.5279, 9.9187) -> (-14.563, 9.9374) construction
  line L587 (-14.5991, 9.9538) -> (-14.6363, 9.9678) construction
  line L588 (-25.4009, 9.9538) -> (-25.437, 9.9374) construction
  line L589 (14.713, 9.9883) -> (14.6743, 9.9793) construction
  line L590 (-25.4721, 9.9187) -> (-25.5058, 9.8977) construction
  line L591 (-14.6363, 9.9678) -> (-14.6743, 9.9793) construction
  line L592 (-25.3637, 9.9678) -> (-25.4009, 9.9538) construction
  line L593 (-24.5, 6.5607) -> (-27.1607, 3.9) construction
  line L594 (-25.437, 9.9374) -> (-25.4721, 9.9187) construction
  line L595 (-25.287, 9.9883) -> (-25.3257, 9.9793) construction
  line L596 (-14.4312, 9.8494) -> (-14.4619, 9.8746) construction
  line L597 (-25.2478, 9.9948) -> (-25.287, 9.9883) construction
  line L598 (-25.1, 10) -> (-25.2083, 9.9987) construction
  line L599 (-25.5978, 9.8222) -> (-26.8786, 8.5414) construction
  line L600 (-14.4619, 9.8746) -> (-14.4942, 9.8977) construction
  line L601 (-14.4942, 9.8977) -> (-14.5279, 9.9187) construction
  line L602 (14.9, 10) -> (14.7917, 9.9987) construction
  line L603 (-30, 3.7001) -> (-30.1999, 3.9) construction
  line L604 (-25.5688, 9.8494) -> (-25.5978, 9.8222) construction
  line L605 (-14.7917, 9.9987) -> (-14.9, 10) construction
  line L606 (14.4619, 9.8746) -> (14.4312, 9.8494) construction
  line L607 (14.4312, 9.8494) -> (14.4022, 9.8222) construction
  line L608 (-15.5, 6.5607) -> (-15.5, 8.2) construction
  line L609 (14.5279, 9.9187) -> (14.4942, 9.8977) construction
  line L610 (14.4942, 9.8977) -> (14.4619, 9.8746) construction
  line L611 (-38.5, 10) -> (-39.5, 10) construction
  line L612 (-14.6743, 9.9793) -> (-14.713, 9.9883) construction
  line L613 (-14.7522, 9.9948) -> (-14.7917, 9.9987) construction
  line L614 (-34.9, 10) -> (-38.5, 10) construction
  line L615 (-34.6743, 9.9793) -> (-34.713, 9.9883) construction
  line L616 (14.4022, 9.8222) -> (13.1214, 8.5414) construction
  line L617 (-34.4022, 9.8222) -> (-34.4312, 9.8494) construction
  line L618 (14.6743, 9.9793) -> (14.6363, 9.9678) construction
  line L619 (14.6363, 9.9678) -> (14.5991, 9.9538) construction
  line L620 (14.5991, 9.9538) -> (14.563, 9.9374) construction
  line L621 (-25.3257, 9.9793) -> (-25.3637, 9.9678) construction
  arc A36 (-13.2628, 8.2) -> (-13.1214, 8.5414) centre (-13.2628, 8.4) ccw construction
  line L622 (-25.5058, 9.8977) -> (-25.5381, 9.8746) construction
  line L623 (14.563, 9.9374) -> (14.5279, 9.9187) construction
  line L624 (-34.4312, 9.8494) -> (-34.4619, 9.8746) construction
  line L625 (-14.713, 9.9883) -> (-14.7522, 9.9948) construction
  line L626 (-13.9, 2.8393) -> (-13.9, 0.207) construction
  line L627 (-35.5, 8.2) -> (-33.2628, 8.2) construction
  line L628 (-34.7522, 9.9948) -> (-34.7917, 9.9987) construction
  line L629 (12.8393, 3.9) -> (10.1999, 3.9) construction
  line L630 (-13.9, -0.207) -> (-13.9, -2.8393) construction
  line L631 (15.5, 8.2) -> (15.5, 6.5607) construction
  line L632 (-33.1214, 8.5414) -> (-34.4022, 9.8222) construction
  line L633 (-13.9, 0.207) -> (-13.693, 0) construction
  line L634 (-34.713, 9.9883) -> (-34.7522, 9.9948) construction
  line L635 (-17.3, 8.2) -> (-17.3, 6.2393) construction
  line L636 (-13.693, 0) -> (-13.9, -0.207) construction
  line L637 (13.9, 0.207) -> (13.9, 2.8393) construction
  line L638 (-34.563, 9.9374) -> (-34.5991, 9.9538) construction
  line L639 (13.2628, 8.2) -> (15.5, 8.2) construction
  line L640 (-15.5, -6.5607) -> (-12.8393, -3.9) construction
  line L641 (-14.9, 10) -> (-25.1, 10) construction
  line L642 (-34.5279, 9.9187) -> (-34.563, 9.9374) construction
  line L643 (-17.3, 6.2393) -> (-13.9, 2.8393) construction
  line L644 (-34.7917, 9.9987) -> (-34.9, 10) construction
  line L645 (15.5, 6.5607) -> (12.8393, 3.9) construction
  arc A37 (-33.2628, 8.2) -> (-33.1214, 8.5414) centre (-33.2628, 8.4) ccw construction
  line L646 (-34.6363, 9.9678) -> (-34.6743, 9.9793) construction
  line L647 (-34.5991, 9.9538) -> (-34.6363, 9.9678) construction
  line L648 (-34.4942, 9.8977) -> (-34.5279, 9.9187) construction
  line L649 (-35.5, 6.5607) -> (-35.5, 8.2) construction
  line L650 (-12.8393, -3.9) -> (-10.1999, -3.9) construction
  arc A38 (13.1214, 8.5414) -> (13.2628, 8.2) centre (13.2628, 8.4) ccw construction
  line L651 (-40, 9.5) -> (-40, 8.5) construction
  arc A39 (-39.5, 10) -> (-40, 9.5) centre (-39.5, 9.5) ccw construction
  line L652 (-22.7, 8.2) -> (-17.3, 8.2) construction
  line L653 (-34.4619, 9.8746) -> (-34.4942, 9.8977) construction
  line L654 (17.3, 8.2) -> (22.7, 8.2) construction
  line L655 (13.9, 2.8393) -> (17.3, 6.2393) construction
  line L656 (25.1, 10) -> (14.9, 10) construction
  line L657 (-39.9883, 4.713) -> (-39.9793, 4.6743) construction
  arc A40 (-38.5414, 3.1214) -> (-38.2, 3.2628) centre (-38.4, 3.2628) ccw construction
  line L658 (-39.9948, 4.7522) -> (-39.9883, 4.713) construction
  line L659 (17.3, 6.2393) -> (17.3, 8.2) construction
  line L660 (-39.9538, 4.5991) -> (-39.9374, 4.563) construction
  line L661 (14.563, -9.9374) -> (14.5991, -9.9538) construction
  line L662 (14.6743, -9.9793) -> (14.713, -9.9883) construction
  line L663 (13.2628, 8.2) -> (15.5, 8.2) construction
  line L664 (15.5, -8.2) -> (13.2628, -8.2) construction
  line L665 (39.9678, 4.6363) -> (39.9793, 4.6743) construction
  line L666 (-22.7, -8.2) -> (-22.7, -6.2393) construction
  line L667 (39.8494, 4.4312) -> (39.8746, 4.4619) construction
  line L668 (14.4022, -9.8222) -> (14.4312, -9.8494) construction
  line L669 (-29.8001, -3.9) -> (-27.1607, -3.9) construction
  line L670 (38.5414, 3.1214) -> (39.8222, 4.4022) construction
  line L671 (39.8222, 4.4022) -> (39.8494, 4.4312) construction
  arc A41 (13.2628, -8.2) -> (13.1214, -8.5414) centre (13.2628, -8.4) ccw construction
  line L672 (39.9374, 4.563) -> (39.9538, 4.5991) construction
  line L673 (-32.8393, -3.9) -> (-30.1999, -3.9) construction
  line L674 (14.4312, -9.8494) -> (14.4619, -9.8746) construction
  line L675 (-32.8393, 3.9) -> (-35.5, 6.5607) construction
  line L676 (39.9538, 4.5991) -> (39.9678, 4.6363) construction
  line L677 (-27.1607, -3.9) -> (-24.5, -6.5607) construction
  line L678 (13.1214, -8.5414) -> (14.4022, -9.8222) construction
  line L679 (-30.1999, -3.9) -> (-30, -3.7001) construction
  line L680 (17.3, -8.2) -> (17.3, -6.2393) construction
  line L681 (17.3, -6.2393) -> (13.9, -2.8393) construction
  line L682 (13.9, -0.207) -> (13.693, 0) construction
  line L683 (14.5279, -9.9187) -> (14.563, -9.9374) construction
  line L684 (14.4942, -9.8977) -> (14.5279, -9.9187) construction
  line L685 (39.8977, 4.4942) -> (39.9187, 4.5279) construction
  line L686 (-30, -3.7001) -> (-29.8001, -3.9) construction
  line L687 (-40, 8.5) -> (-40, 4.8314) construction
  line L688 (39.8746, 4.4619) -> (39.8977, 4.4942) construction
  line L689 (14.7522, -9.9948) -> (14.7917, -9.9987) construction
  line L690 (39.9187, 4.5279) -> (39.9374, 4.563) construction
  line L691 (-24.5, -6.5607) -> (-24.5, -8.2) construction
  line L692 (5.5978, -9.8222) -> (6.8786, -8.5414) construction
  line L693 (-40, 4.8314) -> (-39.9987, 4.7917) construction
  line L694 (-35.5, 8.2) -> (-33.2628, 8.2) construction
  line L695 (-35.5, 6.5607) -> (-35.5, 8.2) construction
  line L696 (34.5991, 9.9538) -> (34.563, 9.9374) construction
  line L697 (5.437, -9.9374) -> (5.4721, -9.9187) construction
  line L698 (5.1, -10) -> (5.2083, -9.9987) construction
  circle A42 centre (10, 0) radius 2.1 construction
  line L699 (5.5688, -9.8494) -> (5.5978, -9.8222) construction
  line L700 (6.1, 0.207) -> (6.307, 0) construction
  line L701 (34.713, 9.9883) -> (34.6743, 9.9793) construction
  line L702 (34.9, 10) -> (34.7917, 9.9987) construction
  line L703 (5.5381, -9.8746) -> (5.5688, -9.8494) construction
  line L704 (34.6363, 9.9678) -> (34.5991, 9.9538) construction
  line L705 (5.2478, -9.9948) -> (5.287, -9.9883) construction
  line L706 (-38.5, 10) -> (-39.5, 10) construction
  line L707 (34.7917, 9.9987) -> (34.7522, 9.9948) construction
  line L708 (4.5, -6.5607) -> (7.1607, -3.9) construction
  line L709 (-34.9, 10) -> (-38.5, 10) construction
  line L710 (5.5058, -9.8977) -> (5.5381, -9.8746) construction
  line L711 (5.4721, -9.9187) -> (5.5058, -9.8977) construction
  line L712 (34.7522, 9.9948) -> (34.713, 9.9883) construction
  line L713 (34.6743, 9.9793) -> (34.6363, 9.9678) construction
  line L714 (9.8001, -3.9) -> (10, -3.7001) construction
  line L715 (5.3257, -9.9793) -> (5.3637, -9.9678) construction
  line L716 (-39.9987, 4.7917) -> (-39.9948, 4.7522) construction
  line L717 (-39.9374, 4.563) -> (-39.9187, 4.5279) construction
  line L718 (-39.8494, 4.4312) -> (-39.8222, 4.4022) construction
  line L719 (14.4312, 9.8494) -> (14.4022, 9.8222) construction
  line L720 (-39.8746, 4.4619) -> (-39.8494, 4.4312) construction
  line L721 (-39.9187, 4.5279) -> (-39.8977, 4.4942) construction
  line L722 (7.1607, -3.9) -> (9.8001, -3.9) construction
  line L723 (-39.9883, 4.713) -> (-39.9793, 4.6743) construction
  line L724 (14.5279, 9.9187) -> (14.4942, 9.8977) construction
  line L725 (10, -3.7001) -> (10.1999, -3.9) construction
  line L726 (6.1, -2.8393) -> (2.7, -6.2393) construction
  line L727 (-39.9538, 4.5991) -> (-39.9374, 4.563) construction
  line L728 (14.4942, 9.8977) -> (14.4619, 9.8746) construction
  line L729 (39.5, 10) -> (38.5, 10) construction
  line L730 (15.5, 8.2) -> (15.5, 6.5607) construction
  line L731 (6.1, 2.8393) -> (6.1, 0.207) construction
  line L732 (40, 8.5) -> (40, 9.5) construction
  arc A43 (40, 9.5) -> (39.5, 10) centre (39.5, 9.5) ccw construction
  line L733 (15.5, 6.5607) -> (12.8393, 3.9) construction
  line L734 (-39.8977, 4.4942) -> (-39.8746, 4.4619) construction
  line L735 (-39.9678, 4.6363) -> (-39.9538, 4.5991) construction
  line L736 (38.5, 10) -> (34.9, 10) construction
  line L737 (-39.9793, 4.6743) -> (-39.9678, 4.6363) construction
  line L738 (5.2083, -9.9987) -> (5.2478, -9.9948) construction
  line L739 (17.3, 6.2393) -> (17.3, 8.2) construction
  line L740 (-39.9948, 4.7522) -> (-39.9883, 4.713) construction
  line L741 (5.287, -9.9883) -> (5.3257, -9.9793) construction
  line L742 (6.307, 0) -> (6.1, -0.207) construction
  line L743 (14.563, 9.9374) -> (14.5279, 9.9187) construction
  line L744 (-39.8222, 4.4022) -> (-38.5414, 3.1214) construction
  line L745 (14.6363, 9.9678) -> (14.5991, 9.9538) construction
  line L746 (-38.2, 5.5) -> (-36.5607, 5.5) construction
  arc A44 (13.1214, 8.5414) -> (13.2628, 8.2) centre (13.2628, 8.4) ccw construction
  line L747 (14.7522, 9.9948) -> (14.713, 9.9883) construction
  line L748 (14.7917, 9.9987) -> (14.7522, 9.9948) construction